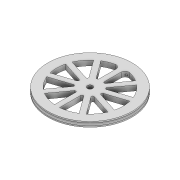
# Autodesk Inventor part: Primary_pulley_V2
Saved by Autodesk Inventor 2022 (Build 260153000, 153)
## iProperties
Created: 2022-07-12
Part Number: Primary_pulley_V2
Material: Generic
Document SubType Name: Modeling
Designer: dell
Density: 1 g/cm^3
Appearance: Default
Mass: 5.02033 g
Surface Area: 47.7091 cm^2
Volume: 5.02033 cm^3
Author: dell
Autodesk Inventor part; units mm, degrees
ref_plane "YZ Plane" through (0, 0, 0) normal (1, 0, 0) x (0, 1, 0)
ref_plane "XZ Plane" through (0, 0, 0) normal (0, 1, 0) x (-1, 0, 0)
sketch "Sketch1" plane through (0, 0, 0) normal (0, 1, 0) x (-1, 0, 0)
  circle A0 centre (0, 0) radius 2.05
  circle A1 centre (0, 0) radius 30
  circle A2 centre (0, -30) radius 2
  point P0 (-1.9989, -29.9333)
  point P1 (1.9989, -29.9333)
  dimension "d2" = 60
  dimension "d0" = 4.1
  dimension "d3" = 4
  constraints: 2 centre point, 2 coincident, 1 vertical alignment, 3 other
  measures "d0" diameter of A0
  measures "d3" diameter of A2
extrude "Extrusion1" add sketch "Sketch1" along normal blind 2 contours A1 A2 picked at (-3.5358, -19.5335)
sketch "Sketch11" plane through (0, 2, 0) normal (0, 1, 0) x (1, 0, 0)
  circle A0 centre (0, 0) radius 2.05 projected
  circle A1 centre (0, 0) radius 26
  line L0 (0, 41.92) -> (0, -41.9867) projected
  line L1 (-42, 0) -> (42, 0) projected
  circle A2 centre (0, 0) radius 5.05
  line L2 (-2, 25.923) -> (-2, -25.923)
  line L3 (2, 25.923) -> (2, -25.923)
  line L4 (-16.8552, 19.7965) -> (13.6191, -22.1477)
  line L5 (-13.6191, 22.1477) -> (16.8552, -19.7965)
  line L6 (-25.2722, 6.1085) -> (24.0362, -9.9127)
  line L7 (-24.0362, 9.9127) -> (25.2722, -6.1085)
  line L8 (-24.0362, -9.9127) -> (25.2722, 6.1085)
  line L9 (-25.2722, -6.1085) -> (24.0362, 9.9127)
  line L10 (-13.6191, -22.1477) -> (16.8552, 19.7965)
  line L11 (-16.8552, -19.7965) -> (13.6191, 22.1477)
  line L12 (2, -25.923) -> (2, 25.923)
  line L13 (-2, -25.923) -> (-2, 25.923)
  line L14 (16.8552, -19.7965) -> (-13.6191, 22.1477)
  line L15 (13.6191, -22.1477) -> (-16.8552, 19.7965)
  line L16 (25.2722, -6.1085) -> (-24.0362, 9.9127)
  line L17 (24.0362, -9.9127) -> (-25.2722, 6.1085)
  line L18 (24.0362, 9.9127) -> (-25.2722, -6.1085)
  line L19 (25.2722, 6.1085) -> (-24.0362, -9.9127)
  line L20 (13.6191, 22.1477) -> (-16.8552, -19.7965)
  line L21 (16.8552, 19.7965) -> (-13.6191, -22.1477)
  point P0 (-2, 4.6371)
  point P1 (2, 4.6371)
  point P2 (2, -4.6371)
  point P3 (-2, -4.6371)
  point P4 (13.6191, -22.1477)
  point P5 (2, -6.1554)
  point P6 (24.0362, -9.9127)
  point P7 (5.2361, -3.8042)
  point P8 (16.8552, -19.7965)
  point P9 (25.2722, 6.1085)
  point P10 (6.4721, 0)
  point P11 (25.2722, -6.1085)
  point P12 (16.8552, 19.7965)
  point P13 (5.2361, 3.8042)
  point P14 (24.0362, 9.9127)
  point P15 (2, 6.1554)
  point P16 (13.6191, 22.1477)
  point P17 (-2, 6.1554)
  point P18 (-5.2361, 3.8042)
  point P19 (-6.4721, 0)
  point P20 (-5.2361, -3.8042)
  point P21 (-2, -6.1554)
  dimension "d76" = 52
  dimension "d81" = 3
  dimension "d87" = 4
  dimension "d88" = 2
  dimension "d94" = 360
  constraints: 40 end point, 4 point on circle, 2 centre point, 2 vertical, 1 coincident, 61 other
  measures "d76" diameter of A1
  measures "d81" radial gap between concentric circles of A0 A2
  measures "d87" distance between parallel lines of L2 L3
  measures "d88" distance from line of point (0, 0) L2
extrude "Extrusion13" cut sketch "Sketch11" against normal blind 10 contours L8 A1 L1 | L1 A1 L7 | L6 A1 L5 | L10 A1 L9 | L3 A1 L11 | L4 A1 L3 | L5 A1 L2 | L2 A1 L10 | L9 A1 L1 | L1 A1 L6 | L7 A1 L4 | L11 A1 L8
ref_plane "Work Plane8" through (-1.9989, 0, -29.9333) normal (-0.6427876, 0, 0.7660444) x (0, 1, 0)
ref_plane "Work Plane9" through (1.9989, 0, -29.9333) normal (0.6427876, 0, 0.7660444) x (0, 1, 0)
sketch "Sketch14" plane through (-1.9989, 0, -29.9333) normal (-0.6427876, 0, 0.7660444) x (0, 1, 0)
  circle A0 centre (0.5, -2.0625) radius 0.75
  line L0 (0, -3.0625) -> (2, -3.0625) projected
  line L1 (2, 0) -> (2, -3.4884) projected
  point P0 (0, -20.772)
  dimension "d103" = 1.5
  dimension "d104" = 1.5
  dimension "d112" = 1
  constraints: 1 centre point
  measures "d103" diameter of A0
  measures "d104" distance from line of L1 A0.centre
  measures "d112" distance from line of L0 A0.centre
sketch "Sketch15" plane through (1.9989, 0, -29.9333) normal (0.6427876, 0, 0.7660444) x (0, 1, 0)
  circle A0 centre (0.5, 2.0625) radius 0.75
  line L0 (0, 3.0625) -> (2, 3.0625) projected
  line L1 (2, 3.4884) -> (2, 0) projected
  point P0 (0, 20.772)
  dimension "d105" = 1.5
  dimension "d106" = 1.5
  dimension "d111" = 1
  constraints: 1 centre point
  measures "d105" diameter of A0
  measures "d106" distance from line of L1 A0.centre
  measures "d111" distance from line of L0 A0.centre
fillet "Fillet4" radius 3 4 edges at (-2, 1, -25.923) (2, 1, -25.923) (1.9989, 1, -29.9333) (-1.9989, 1, -29.9333)
fillet "Fillet5" radius 1 10 edges at (-5.2361, 1, -3.8042) (-6.4721, 1, 0) (-5.2361, 1, 3.8042) (-2, 1, 6.1554) (2, 1, 6.1554) (5.2361, 1, 3.8042) (6.4721, 1, 0) (5.2361, 1, -3.8042) (2, 1, -6.1554) (-2, 1, -6.1554)
extrude "Extrusion14" cut sketch "Sketch15" along normal blind 10
extrude "Extrusion15" cut sketch "Sketch14" along normal blind 10
fillet "Fillet6" radius 1 1 edges at (0, 0.5, -27.9401)
sketch "Sketch16" plane through (0, 0, 0) normal (0, -1, 0) x (1, 0, 0)
  circle A0 centre (0, 0) radius 30
  circle A1 centre (0, 0) radius 33
  arc A2 (-4.2059, -29.7037) -> (-1.5141, -28.6933) centre (-3.7854, -26.7333) ccw projected
  arc A3 (4.2059, -29.7037) -> (-4.2059, -29.7037) centre (0, 0) ccw projected
  arc A4 (1.5141, -28.6933) -> (4.2059, -29.7037) centre (3.7854, -26.7333) ccw projected
  arc A5 (1.5141, -28.6933) -> (-1.5141, -28.6933) centre (0, -30) ccw projected
  arc A6 (-25.2722, 6.1085) -> (-25.2722, -6.1085) centre (0, 0) ccw projected
  line L0 (-25.2722, -6.1085) -> (-9.3992, -0.9511) projected
  arc A7 (-9.3992, -0.9511) -> (-9.3992, 0.9511) centre (-9.7082, 0) ccw projected
  line L1 (-9.3992, 0.9511) -> (-25.2722, 6.1085) projected
  arc A8 (16.8552, -19.7965) -> (24.0362, -9.9127) centre (0, 0) ccw projected
  line L2 (24.0362, -9.9127) -> (8.1631, -4.7553) projected
  arc A9 (8.1631, -4.7553) -> (7.0451, -6.2941) centre (7.8541, -5.7063) ccw projected
  line L3 (7.0451, -6.2941) -> (16.8552, -19.7965) projected
  arc A10 (13.6191, 22.1477) -> (2, 25.923) centre (0, 0) ccw projected
  line L4 (2, 25.923) -> (2, 9.2331) projected
  arc A11 (2, 9.2331) -> (3.809, 8.6453) centre (3, 9.2331) ccw projected
  line L5 (3.809, 8.6453) -> (13.6191, 22.1477) projected
  line L6 (2, -9.2331) -> (2, -22.4499) projected
  arc A12 (2, -22.4499) -> (5.6522, -25.3782) centre (5, -22.4499) ccw projected
  arc A13 (5.6522, -25.3782) -> (13.6191, -22.1477) centre (0, 0) ccw projected
  line L7 (13.6191, -22.1477) -> (3.809, -8.6453) projected
  arc A14 (3.809, -8.6453) -> (2, -9.2331) centre (3, -9.2331) ccw projected
  arc A15 (-16.8552, 19.7965) -> (-24.0362, 9.9127) centre (0, 0) ccw projected
  line L8 (-24.0362, 9.9127) -> (-8.1631, 4.7553) projected
  arc A16 (-8.1631, 4.7553) -> (-7.0451, 6.2941) centre (-7.8541, 5.7063) ccw projected
  line L9 (-7.0451, 6.2941) -> (-16.8552, 19.7965) projected
  arc A17 (-24.0362, -9.9127) -> (-16.8552, -19.7965) centre (0, 0) ccw projected
  line L10 (-16.8552, -19.7965) -> (-7.0451, -6.2941) projected
  arc A18 (-7.0451, -6.2941) -> (-8.1631, -4.7553) centre (-7.8541, -5.7063) ccw projected
  line L11 (-8.1631, -4.7553) -> (-24.0362, -9.9127) projected
  arc A19 (25.2722, -6.1085) -> (25.2722, 6.1085) centre (0, 0) ccw projected
  line L12 (25.2722, 6.1085) -> (9.3992, 0.9511) projected
  arc A20 (9.3992, 0.9511) -> (9.3992, -0.9511) centre (9.7082, 0) ccw projected
  line L13 (9.3992, -0.9511) -> (25.2722, -6.1085) projected
  arc A21 (24.0362, 9.9127) -> (16.8552, 19.7965) centre (0, 0) ccw projected
  line L14 (16.8552, 19.7965) -> (7.0451, 6.2941) projected
  arc A22 (7.0451, 6.2941) -> (8.1631, 4.7553) centre (7.8541, 5.7063) ccw projected
  line L15 (8.1631, 4.7553) -> (24.0362, 9.9127) projected
  arc A23 (-13.6191, -22.1477) -> (-5.6522, -25.3782) centre (0, 0) ccw projected
  arc A24 (-5.6522, -25.3782) -> (-2, -22.4499) centre (-5, -22.4499) ccw projected
  line L16 (-2, -22.4499) -> (-2, -9.2331) projected
  arc A25 (-2, -9.2331) -> (-3.809, -8.6453) centre (-3, -9.2331) ccw projected
  line L17 (-3.809, -8.6453) -> (-13.6191, -22.1477) projected
  line L18 (-2, 9.2331) -> (-2, 25.923) projected
  arc A26 (-2, 25.923) -> (-13.6191, 22.1477) centre (0, 0) ccw projected
  line L19 (-13.6191, 22.1477) -> (-3.809, 8.6453) projected
  arc A27 (-3.809, 8.6453) -> (-2, 9.2331) centre (-3, 9.2331) ccw projected
  circle A28 centre (0, 0) radius 2.05 projected
  arc A29 (4.2059, -29.7037) -> (-4.2059, -29.7037) centre (0, 0) ccw projected
  dimension "d114" = 3
  constraints: 2 centre point, 1 coincident, 1 concentric
  measures "d114" radial gap between concentric circles of A0 A1
extrude "Extrusion16" add sketch "Sketch16" along normal blind 1 contours A0 A4 A5 A2 | A2 A5 A4 A0 | A1
sketch "Sketch18" plane through (0, 2, 0) normal (0, 1, 0) x (1, 0, 0)
  circle A0 centre (0, 0) radius 30
  circle A1 centre (0, 0) radius 33
  arc A2 (-1.5141, 28.6933) -> (-4.2059, 29.7037) centre (-3.7854, 26.7333) ccw projected
  arc A3 (-4.2059, 29.7037) -> (4.2059, 29.7037) centre (0, 0) ccw projected
  arc A4 (4.2059, 29.7037) -> (1.5141, 28.6933) centre (3.7854, 26.7333) ccw projected
  arc A5 (-1.5141, 28.6933) -> (1.5141, 28.6933) centre (0, 30) ccw projected
  arc A6 (-25.2722, 6.1085) -> (-25.2722, -6.1085) centre (0, 0) ccw projected
  line L0 (-25.2722, 6.1085) -> (-9.3992, 0.9511) projected
  arc A7 (-9.3992, -0.9511) -> (-9.3992, 0.9511) centre (-9.7082, 0) ccw projected
  line L1 (-9.3992, -0.9511) -> (-25.2722, -6.1085) projected
  arc A8 (24.0362, 9.9127) -> (16.8552, 19.7965) centre (0, 0) ccw projected
  line L2 (24.0362, 9.9127) -> (8.1631, 4.7553) projected
  arc A9 (7.0451, 6.2941) -> (8.1631, 4.7553) centre (7.8541, 5.7063) ccw projected
  line L3 (7.0451, 6.2941) -> (16.8552, 19.7965) projected
  arc A10 (2, -25.923) -> (13.6191, -22.1477) centre (0, 0) ccw projected
  line L4 (2, -25.923) -> (2, -9.2331) projected
  arc A11 (3.809, -8.6453) -> (2, -9.2331) centre (3, -9.2331) ccw projected
  line L5 (3.809, -8.6453) -> (13.6191, -22.1477) projected
  line L6 (2, 9.2331) -> (2, 22.4499) projected
  arc A12 (5.6522, 25.3782) -> (2, 22.4499) centre (5, 22.4499) ccw projected
  arc A13 (13.6191, 22.1477) -> (5.6522, 25.3782) centre (0, 0) ccw projected
  line L7 (13.6191, 22.1477) -> (3.809, 8.6453) projected
  arc A14 (2, 9.2331) -> (3.809, 8.6453) centre (3, 9.2331) ccw projected
  arc A15 (-24.0362, -9.9127) -> (-16.8552, -19.7965) centre (0, 0) ccw projected
  line L8 (-24.0362, -9.9127) -> (-8.1631, -4.7553) projected
  arc A16 (-7.0451, -6.2941) -> (-8.1631, -4.7553) centre (-7.8541, -5.7063) ccw projected
  line L9 (-7.0451, -6.2941) -> (-16.8552, -19.7965) projected
  arc A17 (-16.8552, 19.7965) -> (-24.0362, 9.9127) centre (0, 0) ccw projected
  line L10 (-16.8552, 19.7965) -> (-7.0451, 6.2941) projected
  arc A18 (-8.1631, 4.7553) -> (-7.0451, 6.2941) centre (-7.8541, 5.7063) ccw projected
  line L11 (-8.1631, 4.7553) -> (-24.0362, 9.9127) projected
  arc A19 (25.2722, -6.1085) -> (25.2722, 6.1085) centre (0, 0) ccw projected
  line L12 (25.2722, -6.1085) -> (9.3992, -0.9511) projected
  arc A20 (9.3992, 0.9511) -> (9.3992, -0.9511) centre (9.7082, 0) ccw projected
  line L13 (9.3992, 0.9511) -> (25.2722, 6.1085) projected
  arc A21 (16.8552, -19.7965) -> (24.0362, -9.9127) centre (0, 0) ccw projected
  line L14 (16.8552, -19.7965) -> (7.0451, -6.2941) projected
  arc A22 (8.1631, -4.7553) -> (7.0451, -6.2941) centre (7.8541, -5.7063) ccw projected
  line L15 (8.1631, -4.7553) -> (24.0362, -9.9127) projected
  arc A23 (-5.6522, 25.3782) -> (-13.6191, 22.1477) centre (0, 0) ccw projected
  arc A24 (-2, 22.4499) -> (-5.6522, 25.3782) centre (-5, 22.4499) ccw projected
  line L16 (-2, 22.4499) -> (-2, 9.2331) projected
  arc A25 (-3.809, 8.6453) -> (-2, 9.2331) centre (-3, 9.2331) ccw projected
  line L17 (-3.809, 8.6453) -> (-13.6191, 22.1477) projected
  line L18 (-2, -9.2331) -> (-2, -25.923) projected
  arc A26 (-13.6191, -22.1477) -> (-2, -25.923) centre (0, 0) ccw projected
  line L19 (-13.6191, -22.1477) -> (-3.809, -8.6453) projected
  arc A27 (-2, -9.2331) -> (-3.809, -8.6453) centre (-3, -9.2331) ccw projected
  circle A28 centre (0, 0) radius 2.05 projected
  arc A29 (-4.2059, 29.7037) -> (4.2059, 29.7037) centre (0, 0) ccw projected
  dimension "d117" = 3
  constraints: 2 centre point, 1 coincident, 1 concentric
  measures "d117" radial gap between concentric circles of A0 A1
extrude "Extrusion17" add sketch "Sketch18" along normal blind 1 contours A0 A2 A5 A4 | A4 A5 A2 A0 | A1
body "Solid1"
